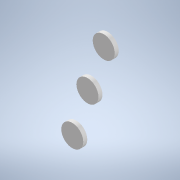
# Autodesk Inventor part: WheelCover
Saved by Autodesk Inventor 2020 (Build 240168000, 168)
## iProperties
Created: 2020-01-19
Part Number: WheelCover
Material: Generic
Document SubType Name: Modeling
Designer: srini
Density: 1 g/cm^3
Appearance: Default
Author: srini
Autodesk Inventor part; units mm, degrees
ref_plane "YZ Plane" through (0, 0, 0) normal (1, 0, 0) x (0, 1, 0)
ref_plane "XZ Plane" through (0, 0, 0) normal (0, 1, 0) x (-1, 0, 0)
sketch "Sketch1" plane through (0, 0, 0) normal (0, 0, 1) x (1, 0, 0)
  circle A0 centre (66.294, 0) radius 66.3424 projected
  circle A1 centre (-31.9923, -278.2214) radius 66.3424 projected
  circle A2 centre (-123.5448, -558.7308) radius 66.3424 projected
  point P0 (0, 0)
ref_plane "Work Plane1" through (-256.2384, -691.4245, -24.2951) normal (0, 0, -1) x (-0.3658, 0.9307, 0)
extrude "Extrusion1" add sketch "Sketch1" against normal up to surface (24.2951 mm away)
body "Solid1"
